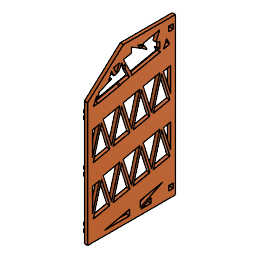
side-panel-right (Autodesk Fusion 360 design; units mm, degrees)
part number: 2026-08-18-20-49-11-243
Autodesk Fusion 360 part; units mm, degrees
sketch "Sketch1" plane through (0, 0, 0) normal (1, 0, 0) x (0, 0, -1)
  line L0 (0, 15) -> (0, 150)
  line L1 (0, 150) -> (-240, 150)
  line L2 (-240, 150) -> (-240, 70)
  line L3 (-240, 70) -> (-190, 15)
  line L4 (-190, 15) -> (0, 15)
extrude "Extrude1" add sketch "Sketch1" along normal blind 5 from surface at 6 makes body 1
sketch "Sketch2" plane through (0, 0, 0) normal (1, 0, 0) x (0, 0, -1)
  line L0 (-9, 20) -> (-35.5696, 145)
  line L1 (-35.5696, 145) -> (-41.5696, 145)
  line L2 (-41.5696, 145) -> (-15, 20)
  line L3 (-15, 20) -> (-9, 20)
extrude "Extrude2" add sketch "Sketch2" along normal blind 6 separate body makes body 2
sketch "Sketch3" plane through (0, 0, 0) normal (1, 0, 0) x (0, 0, -1)
  line L0 (-18.2, 20) -> (-44.7696, 145)
  line L1 (-44.7696, 145) -> (-49.7696, 145)
  line L2 (-49.7696, 145) -> (-23.2, 20)
  line L3 (-23.2, 20) -> (-18.2, 20)
extrude "Extrude3" add sketch "Sketch3" along normal blind 6 separate body makes body 3
sketch "Sketch4" plane through (0, 0, 0) normal (1, 0, 0) x (0, 0, -1)
  line L0 (-16.2753, 26) -> (-17.2753, 28)
  line L1 (-17.2753, 28) -> (-18.3381, 31)
  line L2 (-18.3381, 31) -> (-17.7632, 33)
  line L3 (-17.7632, 33) -> (-16.2753, 26)
extrude "Extrude4" add sketch "Sketch4" along normal blind 6 separate body makes body 4
sketch "Sketch5" plane through (0, 0, 0) normal (1, 0, 0) x (0, 0, -1)
  line L0 (-84, 20) -> (-110.5696, 145)
  line L1 (-110.5696, 145) -> (-116.5696, 145)
  line L2 (-116.5696, 145) -> (-90, 20)
  line L3 (-90, 20) -> (-84, 20)
extrude "Extrude5" add sketch "Sketch5" along normal blind 6 separate body makes body 5
sketch "Sketch6" plane through (0, 0, 0) normal (1, 0, 0) x (0, 0, -1)
  line L0 (-93.2, 20) -> (-119.7696, 145)
  line L1 (-119.7696, 145) -> (-124.7696, 145)
  line L2 (-124.7696, 145) -> (-98.2, 20)
  line L3 (-98.2, 20) -> (-93.2, 20)
extrude "Extrude6" add sketch "Sketch6" along normal blind 6 separate body makes body 6
sketch "Sketch7" plane through (0, 0, 0) normal (1, 0, 0) x (0, 0, -1)
  line L0 (-91.2753, 26) -> (-92.2753, 28)
  line L1 (-92.2753, 28) -> (-93.3381, 31)
  line L2 (-93.3381, 31) -> (-92.7632, 33)
  line L3 (-92.7632, 33) -> (-91.2753, 26)
extrude "Extrude7" add sketch "Sketch7" along normal blind 6 separate body makes body 7
sketch "Sketch8" plane through (0, 0, 0) normal (1, 0, 0) x (0, 0, -1)
  line L0 (-159, 20) -> (-185.5696, 145)
  line L1 (-185.5696, 145) -> (-191.5696, 145)
  line L2 (-191.5696, 145) -> (-165, 20)
  line L3 (-165, 20) -> (-159, 20)
extrude "Extrude8" add sketch "Sketch8" along normal blind 6 separate body makes body 8
sketch "Sketch9" plane through (0, 0, 0) normal (1, 0, 0) x (0, 0, -1)
  line L0 (-168.2, 20) -> (-194.7696, 145)
  line L1 (-194.7696, 145) -> (-199.7696, 145)
  line L2 (-199.7696, 145) -> (-173.2, 20)
  line L3 (-173.2, 20) -> (-168.2, 20)
extrude "Extrude9" add sketch "Sketch9" along normal blind 6 separate body makes body 9
sketch "Sketch10" plane through (0, 0, 0) normal (1, 0, 0) x (0, 0, -1)
  line L0 (-166.2753, 26) -> (-167.2753, 28)
  line L1 (-167.2753, 28) -> (-168.3381, 31)
  line L2 (-168.3381, 31) -> (-167.7632, 33)
  line L3 (-167.7632, 33) -> (-166.2753, 26)
extrude "Extrude10" add sketch "Sketch10" along normal blind 6 separate body makes body 10
combine "Combine1" operation add target body 1 tool bodies 2 3 4 5 6 7 8 9 10
sketch "Sketch11" plane through (0, 0, 0) normal (1, 0, 0) x (0, 0, -1)
  line L0 (-10.5, 139.5) -> (-10.5, 146.5)
  line L1 (-10.5, 146.5) -> (-17.5, 146.5)
  line L2 (-17.5, 146.5) -> (-17.5, 139.5)
  line L3 (-17.5, 139.5) -> (-10.5, 139.5)
extrude "Extrude11" cut sketch "Sketch11" along normal blind 30 from surface at -2 bodies 1
sketch "Sketch12" plane through (0, 0, 0) normal (1, 0, 0) x (0, 0, -1)
  line L0 (-222.5, 139.5) -> (-222.5, 146.5)
  line L1 (-222.5, 146.5) -> (-229.5, 146.5)
  line L2 (-229.5, 146.5) -> (-229.5, 139.5)
  line L3 (-229.5, 139.5) -> (-222.5, 139.5)
extrude "Extrude12" cut sketch "Sketch12" along normal blind 30 from surface at -2 bodies 1
sketch "Sketch13" plane through (0, 0, 0) normal (1, 0, 0) x (0, 0, -1)
  line L0 (-31.0484, 23.6788) -> (-36.4457, 49.0712)
  line L1 (-36.4457, 49.0712) -> (-77.3478, 36.375)
  line L2 (-77.3478, 36.375) -> (-31.0484, 23.6788)
  line L3 (-37.5845, 54.4288) -> (-42.9818, 79.8212)
  line L4 (-42.9818, 79.8212) -> (-83.8839, 67.125)
  line L5 (-83.8839, 67.125) -> (-37.5845, 54.4288)
  line L6 (-44.1206, 85.1788) -> (-49.5179, 110.5712)
  line L7 (-49.5179, 110.5712) -> (-90.42, 97.875)
  line L8 (-90.42, 97.875) -> (-44.1206, 85.1788)
  line L9 (-50.6567, 115.9288) -> (-56.054, 141.3212)
  line L10 (-56.054, 141.3212) -> (-96.9561, 128.625)
  line L11 (-96.9561, 128.625) -> (-50.6567, 115.9288)
  line L12 (-80.9836, 39.0538) -> (-86.3809, 64.4462)
  line L13 (-86.3809, 64.4462) -> (-40.0815, 51.75)
  line L14 (-40.0815, 51.75) -> (-80.9836, 39.0538)
  line L15 (-87.5197, 69.8038) -> (-92.917, 95.1962)
  line L16 (-92.917, 95.1962) -> (-46.6176, 82.5)
  line L17 (-46.6176, 82.5) -> (-87.5197, 69.8038)
  line L18 (-94.0558, 100.5538) -> (-99.4532, 125.9462)
  line L19 (-99.4532, 125.9462) -> (-53.1537, 113.25)
  line L20 (-53.1537, 113.25) -> (-94.0558, 100.5538)
  line L21 (-38.7362, 22.5992) -> (-75.0606, 22.5992)
  line L22 (-75.0606, 22.5992) -> (-77.3089, 33.1766)
  line L23 (-77.3089, 33.1766) -> (-38.7362, 22.5992)
  line L24 (-63.6735, 142.48) -> (-100.8141, 142.48)
  line L25 (-100.8141, 142.48) -> (-98.5153, 131.6649)
  line L26 (-98.5153, 131.6649) -> (-63.6735, 142.48)
  line L27 (-106.0484, 23.6788) -> (-111.4457, 49.0712)
  line L28 (-111.4457, 49.0712) -> (-152.3478, 36.375)
  line L29 (-152.3478, 36.375) -> (-106.0484, 23.6788)
  line L30 (-112.5845, 54.4288) -> (-117.9818, 79.8212)
  line L31 (-117.9818, 79.8212) -> (-158.8839, 67.125)
  line L32 (-158.8839, 67.125) -> (-112.5845, 54.4288)
  line L33 (-119.1206, 85.1788) -> (-124.5179, 110.5712)
  line L34 (-124.5179, 110.5712) -> (-165.42, 97.875)
  line L35 (-165.42, 97.875) -> (-119.1206, 85.1788)
  line L36 (-125.6567, 115.9288) -> (-131.054, 141.3212)
  line L37 (-131.054, 141.3212) -> (-171.9561, 128.625)
  line L38 (-171.9561, 128.625) -> (-125.6567, 115.9288)
  line L39 (-155.9836, 39.0538) -> (-161.3809, 64.4462)
  line L40 (-161.3809, 64.4462) -> (-115.0815, 51.75)
  line L41 (-115.0815, 51.75) -> (-155.9836, 39.0538)
  line L42 (-162.5197, 69.8038) -> (-167.917, 95.1962)
  line L43 (-167.917, 95.1962) -> (-121.6176, 82.5)
  line L44 (-121.6176, 82.5) -> (-162.5197, 69.8038)
  line L45 (-169.0558, 100.5538) -> (-174.4532, 125.9462)
  line L46 (-174.4532, 125.9462) -> (-128.1537, 113.25)
  line L47 (-128.1537, 113.25) -> (-169.0558, 100.5538)
  line L48 (-113.7362, 22.5992) -> (-150.0606, 22.5992)
  line L49 (-150.0606, 22.5992) -> (-152.3089, 33.1766)
  line L50 (-152.3089, 33.1766) -> (-113.7362, 22.5992)
  line L51 (-138.6735, 142.48) -> (-175.8141, 142.48)
  line L52 (-175.8141, 142.48) -> (-173.5153, 131.6649)
  line L53 (-173.5153, 131.6649) -> (-138.6735, 142.48)
  line L54 (-180.386, 24.1097) -> (-182.3321, 33.2653)
  line L55 (-182.3321, 33.2653) -> (-191.5717, 28.6875)
  line L56 (-191.5717, 28.6875) -> (-180.386, 24.1097)
  line L57 (-183.654, 39.4847) -> (-185.6001, 48.6403)
  line L58 (-185.6001, 48.6403) -> (-194.8398, 44.0625)
  line L59 (-194.8398, 44.0625) -> (-183.654, 39.4847)
  line L60 (-185.3055, 36.375) -> (-196.4912, 40.9528)
  line L61 (-196.4912, 40.9528) -> (-194.5451, 31.7972)
  line L62 (-194.5451, 31.7972) -> (-185.3055, 36.375)
  line L63 (-186.9221, 54.8597) -> (-192.1362, 79.3903)
  line L64 (-192.1362, 79.3903) -> (-216.8918, 67.125)
  line L65 (-216.8918, 67.125) -> (-186.9221, 54.8597)
  line L66 (-193.4582, 85.6097) -> (-198.6724, 110.1403)
  line L67 (-198.6724, 110.1403) -> (-223.428, 97.875)
  line L68 (-223.428, 97.875) -> (-193.4582, 85.6097)
  line L69 (-199.9943, 116.3597) -> (-201.9404, 125.5153)
  line L70 (-201.9404, 125.5153) -> (-211.18, 120.9375)
  line L71 (-211.18, 120.9375) -> (-199.9943, 116.3597)
  line L72 (-203.2624, 131.7347) -> (-205.2085, 140.8903)
  line L73 (-205.2085, 140.8903) -> (-214.4481, 136.3125)
  line L74 (-214.4481, 136.3125) -> (-203.2624, 131.7347)
  line L75 (-216.5972, 54.8597) -> (-218.5433, 64.0153)
  line L76 (-218.5433, 64.0153) -> (-207.3576, 59.4375)
  line L77 (-207.3576, 59.4375) -> (-216.5972, 54.8597)
  line L78 (-197.8132, 47.1722) -> (-199.7593, 56.3278)
  line L79 (-199.7593, 56.3278) -> (-188.5736, 51.75)
  line L80 (-188.5736, 51.75) -> (-197.8132, 47.1722)
  line L81 (-213.6238, 51.75) -> (-204.3842, 56.3278)
  line L82 (-204.3842, 56.3278) -> (-202.4381, 47.1722)
  line L83 (-202.4381, 47.1722) -> (-213.6238, 51.75)
  line L84 (-219.8653, 70.2347) -> (-225.0794, 94.7653)
  line L85 (-225.0794, 94.7653) -> (-195.1097, 82.5)
  line L86 (-195.1097, 82.5) -> (-219.8653, 70.2347)
  line L87 (-226.4014, 100.9847) -> (-231.6155, 125.5153)
  line L88 (-231.6155, 125.5153) -> (-201.6458, 113.25)
  line L89 (-201.6458, 113.25) -> (-226.4014, 100.9847)
  line L90 (-7.4997, 41.3524) -> (-7.4997, 79.3238)
  line L91 (-7.4997, 79.3238) -> (-16.0293, 79.3238)
  line L92 (-16.0293, 79.3238) -> (-7.4997, 41.3524)
  line L93 (-7.7256, 97.1983) -> (-7.7256, 112.4009)
  line L94 (-7.7256, 112.4009) -> (-15.0147, 112.4009)
  line L95 (-15.0147, 112.4009) -> (-7.7256, 97.1983)
  line L96 (-10.4709, 95.9903) -> (-19.5534, 95.9903)
  line L97 (-19.5534, 95.9903) -> (-26.7865, 130.0194)
  line L98 (-26.7865, 130.0194) -> (-10.4709, 95.9903)
  line L99 (-181.1006, 31.0194) -> (-188.5277, 65.9611)
  line L100 (-188.5277, 65.9611) -> (-191.9491, 31.0194)
  line L101 (-191.9491, 31.0194) -> (-181.1006, 31.0194)
  line L102 (-191.1748, 72.6899) -> (-212.3291, 72.6899)
  line L103 (-212.3291, 72.6899) -> (-195.0983, 32.6201)
  line L104 (-195.0983, 32.6201) -> (-191.1748, 72.6899)
  line L105 (-192.5, 82.4034) -> (-202.0204, 127.1932)
  line L106 (-202.0204, 127.1932) -> (-230.4393, 82.4034)
  line L107 (-230.4393, 82.4034) -> (-192.5, 82.4034)
  line L108 (-206.5204, 125.9619) -> (-215.9652, 125.9619)
  line L109 (-215.9652, 125.9619) -> (-228.0207, 92.0761)
  line L110 (-228.0207, 92.0761) -> (-206.5204, 125.9619)
extrude "Extrude13" cut sketch "Sketch13" along normal blind 9 from surface at 4 bodies 1
named bodies: "Тело"
